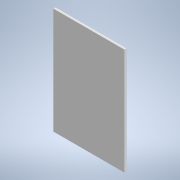
# Autodesk Inventor part: box side
Saved by Autodesk Inventor 2020 (Build 240168000, 168)
## iProperties
Created: 2020-12-15
Part Number: box side
Material: Generic
Document SubType Name: Modeling
Designer: moham
Density: 1 g/cm^3
Appearance: Default
Author: moham
Autodesk Inventor part; units mm, degrees
ref_plane "YZ Plane" through (0, 0, 0) normal (1, 0, 0) x (0, 1, 0)
ref_plane "XZ Plane" through (0, 0, 0) normal (0, 1, 0) x (-1, 0, 0)
ref_plane "XY Plane" through (0, 0, 0) normal (0, 0, 1) x (1, 0, 0)
sketch "Sketch1" plane through (0, 0, 0) normal (0, 0, 1) x (1, 0, 0)
  line L0 (-50, 100) -> (100, 100)
  line L1 (-50, 100) -> (-50, -50)
  line L2 (-50, -50) -> (100, -50)
  line L3 (100, -50) -> (100, 100)
  line L4 (-50, 25) -> (0, 0)
  dimension "d0" = 150
  dimension "d1" = 150
  dimension "d2" = 50
  constraints: 10 end point, 2 perpendicular, 1 horizontal, 1 midpoint, 1 vertical
  measures "d0" distance of L0.start L0.end
  measures "d1" distance of L0.start L1.end
  measures "d2" distance from line of L1 L4.end
sketch "Sketch2" plane through (0, 0, 0) normal (0, 0, 1) x (1, 0, 0)
  point P0 (0, 0)
extrude "Extrusion1" add sketch "Sketch1" along normal blind 3
body "Solid1"
